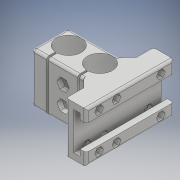
# Autodesk Inventor part: CarroXY - Carro V2
Saved by Autodesk Inventor 2017 (Build 210142000, 142)
## iProperties
Created: 2020-08-15
Part Number: CarroXY - Carro V2
Material: Generic
Document SubType Name: Modeling
Designer: ale
Density: 1 g/cm^3
Appearance: Default
Author: ale
Autodesk Inventor part; units mm, degrees
ref_plane "YZ Plane" through (0, 0, 0) normal (1, 0, 0) x (0, 1, 0)
ref_plane "XZ Plane" through (0, 0, 0) normal (0, 1, 0) x (-1, 0, 0)
ref_plane "XY Plane" through (0, 0, 0) normal (0, 0, 1) x (1, 0, 0)
sketch "Sketch1" plane through (0, 0, 0) normal (0, 0, 1) x (1, 0, 0)
  arc A0 (-11.7683, -9.9732) -> (-13.2317, -9.9732) centre (-12.5, 0) ccw
  arc A1 (13.2317, -9.9732) -> (11.7683, -9.9732) centre (12.5, 0) ccw
  line L0 (23, -17) -> (23, 12)
  line L1 (23, 12) -> (-25, 12)
  line L2 (-25, 12) -> (-25, -17)
  line L3 (-13.2317, -9.9732) -> (-13.2317, -17)
  line L4 (-11.7683, -9.9732) -> (-11.7683, -17)
  line L5 (11.7683, -9.9732) -> (11.7683, -17)
  line L6 (13.2317, -9.9732) -> (13.2317, -17)
  line L7 (13.2317, -17) -> (23, -17)
  line L8 (-25, -17) -> (-13.2317, -17)
  line L9 (-11.7683, -17) -> (11.7683, -17)
  line L10 (-35.4015, 0) -> (35.4015, 0)
  line L11 (0, -27.2768) -> (0, 27.2768)
  point P0 (0, 0)
  point P1 (0, 0)
  point P2 (0, 0)
  dimension "d2" = 20
  dimension "d3" = 20
  dimension "d106" = 17
  dimension "d107" = 17
  dimension "d108" = 17
  dimension "d110" = 12.5
  dimension "d111" = 12.5
  dimension "d113" = 23
  dimension "d114" = 25
  constraints: 24 end point, 4 point on circle, 3 horizontal, 2 centre point, 2 coincident, 2 midpoint, 2 point on line, 1 parallel, 1 vertical
  measures "d2" diameter of A0
  measures "d3" diameter of A1
  measures "d106" distance between parallel lines of L7 L10
  measures "d107" distance between parallel lines of L9 L10
  measures "d108" distance between parallel lines of L8 L10
  measures "d110" distance from line of A1.centre L11
  measures "d111" distance from line of A0.centre L11
  measures "d113" distance between parallel lines of L0 L11
  measures "d114" distance between parallel lines of L2 L11
extrude "Extrusion2" add sketch "Sketch1" along normal blind 40 contours A0 L10 L11 L9 L4 | A0 L10 L2 L1 L11 | A0 L3 L8 L2 L10 | L11 L1 L0 L10 A1 | L10 A1 L5 L9 L11 | L10 L0 L7 L6 A1
sketch "Sketch3" plane through (23, -17, 0) normal (1, 0, 0) x (0, 0, -1)
  line L0 (-40, 49.5) -> (0, 49.5)
  line L1 (0, 49.5) -> (0, -20.5)
  line L2 (0, -20.5) -> (-40, -20.5)
  line L3 (-40, -20.5) -> (-40, 49.5)
  line L4 (-40, 49.5) -> (0, -20.5) construction
  line L5 (0, 49.5) -> (-40, -20.5) construction
  line L6 (0, 29) -> (-40, 29) projected
  line L7 (-20, 29) -> (-20, 0)
  line L8 (0, 0) -> (-40, 0) projected
  line L9 (-40, 0) -> (-40, 29) projected
  line L10 (-40, 14.5) -> (0, 14.5)
  line L11 (0, 29) -> (0, 0) projected
  point P0 (0, 17)
  point P1 (-20, 14.5)
  point P2 (-20, 14.5)
  dimension "d18" = 40
  dimension "d19" = 70
  constraints: 16 end point, 8 midpoint, 2 parallel, 1 horizontal, 1 perpendicular
  measures "d18" distance of L1.end L2.end
  measures "d19" distance between parallel lines of L2 L0
extrude "Extrusion3" add sketch "Sketch3" along normal blind 6
sketch "Sketch13" plane through (-25, 12, 40) normal (0, 1, 0) x (1, 0, 0)
  line L0 (25, 40) -> (25, 0)
  line L1 (13.2317, 0) -> (36.7683, 0) projected
  line L2 (25, 40) -> (65, 40) construction
  line L3 (25, 20) -> (32.3928, 20)
  line L4 (25, 27.5) -> (32.3928, 27.5)
  line L5 (25, 12.5) -> (32.3928, 12.5)
  dimension "d83" = 90
  dimension "d84" = 7.5
  dimension "d85" = 7.5
  constraints: 10 end point, 2 coincident, 2 horizontal, 2 midpoint, 2 parallel, 1 perpendicular
  measures "d83" angle of L0 L2
  measures "d84" distance between parallel lines of L3 L4
  measures "d85" distance between parallel lines of L3 L5
hole "Hole5" at (0, 12, 12.5) at (0, 12, 27.5) direction (0, -1, 0) diameter 4.5 end through all counterbore diameter 10 counterbore depth 3
sketch "Sketch14" plane through (-11.7683, -17, 0) normal (0, -1, 0) x (1, 0, 0)
  circle A0 centre (11.7683, 12.5) radius 2.25 projected
  circle A1 centre (11.7683, 12.5) radius 5 projected
  line L0 (16.7683, 12.5) -> (14.2683, 8.1699)
  line L1 (14.2683, 8.1699) -> (9.2683, 8.1699)
  line L2 (9.2683, 8.1699) -> (6.7683, 12.5)
  line L3 (6.7683, 12.5) -> (9.2683, 16.8301)
  line L4 (9.2683, 16.8301) -> (14.2683, 16.8301)
  line L5 (14.2683, 16.8301) -> (16.7683, 12.5)
  circle A2 centre (11.7683, 27.5) radius 2.25 projected
  circle A3 centre (11.7683, 27.5) radius 5 projected
  line L6 (9.2683, 31.8301) -> (14.2683, 31.8301)
  line L7 (14.2683, 31.8301) -> (16.7683, 27.5)
  line L8 (16.7683, 27.5) -> (14.2683, 23.1699)
  line L9 (14.2683, 23.1699) -> (9.2683, 23.1699)
  line L10 (9.2683, 23.1699) -> (6.7683, 27.5)
  line L11 (6.7683, 27.5) -> (9.2683, 31.8301)
  point P0 (11.7683, 0)
  constraints: 24 end point, 2 coincident, 1 horizontal alignment, 29 other
extrude "Extrusion11" cut sketch "Sketch14" against normal blind 4 contours L0 L1 L2 L3 L4 L5 | L8 L9 L10 L11 L6 L7
sketch "Sketch16" plane through (23, -37.5, 0) normal (0, -1, 0) x (1, 0, 0)
  line L0 (6, 40) -> (6, 0) projected
  line L1 (6, 0) -> (6, 5)
  line L2 (6, 5) -> (11, 5)
  line L3 (11, 5) -> (11, 10)
  line L4 (11, 10) -> (16, 10)
  line L5 (16, 10) -> (16, 0)
  line L6 (16, 0) -> (6, 0)
  line L7 (6, 20) -> (15.5722, 20)
  line L8 (6, 0) -> (6, 40)
  line L9 (6, 40) -> (6, 35)
  line L10 (6, 35) -> (11, 35)
  line L11 (11, 35) -> (11, 30)
  line L12 (11, 30) -> (16, 30)
  line L13 (16, 30) -> (16, 40)
  line L14 (16, 40) -> (6, 40)
  point P0 (-23, 0)
  dimension "d95" = 5
  dimension "d96" = 5
  dimension "d97" = 5
  dimension "d98" = 5
  constraints: 28 end point, 7 symmetric about line, 5 perpendicular, 2 point on line, 1 horizontal, 1 midpoint
  measures "d95" distance of L0.end L1.end
  measures "d96" distance of L1.end L2.end
  measures "d97" distance of L2.end L3.end
  measures "d98" distance of L3.end L4.end
extrude "Extrusion12" add sketch "Sketch16" against normal blind 70
sketch "Sketch10" plane through (-25, -17, 0) normal (-1, 0, 0) x (0, 0, 1)
  line L0 (0, 0) -> (40, 0) projected
  line L1 (20, 0) -> (20, 29)
  line L2 (0, 29) -> (40, 29) projected
  point P0 (0, 17)
  point P1 (35.2144, 3.7)
  point P2 (4.7856, 3.7)
  dimension "d61" = 3.7
  constraints: 2 end point, 2 midpoint, 1 symmetric about line
  measures "d61" distance from line of point (35.214, 3.7) L0
hole "Hole3" at (-25, -13.3, 35.2144) at (-25, -13.3, 4.7856) direction (1, 0, 0) diameter 4.5 end through all
sketch "Sketch17" plane through (39, -37.5, 10) normal (1, 0, 0) x (0, 0, -1)
  circle A0 centre (5.2144, 24.2) radius 2.25 projected
  line L0 (5, 0) -> (5, 70) projected
  line L1 (5, 27.7) -> (8.1383, 26.1357)
  line L2 (8.1383, 26.1357) -> (8.3527, 22.6357)
  line L3 (8.3527, 22.6357) -> (5.4289, 20.7)
  line L4 (5.4289, 20.7) -> (2.2906, 22.2643)
  line L5 (2.2906, 22.2643) -> (2.0761, 25.7643)
  line L6 (2.0761, 25.7643) -> (5, 27.7)
  circle A1 centre (-25.2144, 24.2) radius 2.25 projected
  line L7 (-25, 70) -> (-25, 26.4398) projected
  line L8 (-25, 27.7) -> (-22.0761, 25.7643)
  line L9 (-22.0761, 25.7643) -> (-22.2906, 22.2643)
  line L10 (-22.2906, 22.2643) -> (-25.4289, 20.7)
  line L11 (-25.4289, 20.7) -> (-28.3527, 22.6357)
  line L12 (-28.3527, 22.6357) -> (-28.1383, 26.1357)
  line L13 (-28.1383, 26.1357) -> (-25, 27.7)
  point P0 (10, 37.5)
  point P1 (5.2144, 24.2)
  point P2 (-25.2144, 24.2)
  dimension "d101" = 7
  dimension "d102" = 7
  constraints: 24 end point, 2 coincident, 2 point on line, 27 other
  measures "d101" vertical distance of L1.start L3.end
  measures "d102" vertical distance of L8.start L10.end
extrude "Extrusion13" cut sketch "Sketch17" against normal blind 20 contours A0 L0 L1 L2 L3 L4 | A0 L0 L4 L5 L6 | L8 L9 L10 L11 L12 L13
fillet "Fillet2" radius 2 20 edges at (-25, -17, 20) (-19.1159, -17, 0) (0, -17, 0) (18.1159, -17, 0) (-1, 12, 0) (-25, -2.5, 0) (-25, 12, 20) (-1, 12, 40) (-25, -2.5, 40) (-19.1159, -17, 40) (0, -17, 40) (18.1159, -17, 40) (23, -37.5, 20) (39, -37.5, 5) (39, -37.5, 35) (39, -2.5, 0) (39, -2.5, 40) (23, 32.5, 20) (39, 32.5, 35) (39, 32.5, 5)
sketch "Sketch18" plane through (23, -17, 0) normal (-1, 0, 0) x (0, 0, 1)
  line L0 (40, -18.5) -> (40, 2) projected
  line L1 (2, 0) -> (38, 0) projected
  line L2 (40, -18.5) -> (0, -18.5) projected
  line L3 (20, -18.5) -> (20, -3.6839)
  line L4 (40, 2) -> (40, 27) projected
  line L5 (40, 14.5) -> (0, 14.5)
  point P0 (0, 17)
  point P1 (34.5, -10.25)
  point P2 (5.5, -10.25)
  point P3 (34.5, 39.25)
  point P4 (5.5, 39.25)
  dimension "d119" = 5.5
  dimension "d120" = 10.25
  constraints: 4 end point, 3 symmetric about line, 2 midpoint, 1 horizontal, 1 vertical
  measures "d119" distance from line of L0 point (34.5, -10.25)
  measures "d120" distance from line of L1 point (34.5, -10.25)
chamfer "Chamfer2" distance 7 angle 45 6 edges at (23, -17, 20) (23, -16.4142, 39.4142) (23, -16.4142, 0.5858) (23, 12, 20) (23, 11.4142, 39.4142) (23, 11.4142, 0.5858)
hole "Hole6" at (23, -27.25, 34.5) at (23, -27.25, 5.5) at (23, 22.25, 34.5) at (23, 22.25, 5.5) direction (1, 0, 0) diameter 4.5 end through all
sketch "Sketch19" plane through (39, -35.5, 10) normal (1, 0, 0) x (0, 0, -1)
  circle A0 centre (4.5, 8.25) radius 2.25 projected
  line L0 (4.5, 11.75) -> (7.5311, 10)
  line L1 (7.5311, 10) -> (7.5311, 6.5)
  line L2 (7.5311, 6.5) -> (4.5, 4.75)
  line L3 (4.5, 4.75) -> (1.4689, 6.5)
  line L4 (1.4689, 6.5) -> (1.4689, 10)
  line L5 (1.4689, 10) -> (4.5, 11.75)
  line L6 (-25, -2) -> (5, -2) projected
  line L7 (-10, -2) -> (-10, 68)
  circle A1 centre (-24.5, 8.25) radius 2.25
  line L8 (-24.5, 11.75) -> (-27.5311, 10)
  line L9 (-27.5311, 10) -> (-27.5311, 6.5)
  line L10 (-27.5311, 6.5) -> (-24.5, 4.75)
  line L11 (-24.5, 4.75) -> (-21.4689, 6.5)
  line L12 (-21.4689, 6.5) -> (-21.4689, 10)
  line L13 (-21.4689, 10) -> (-24.5, 11.75)
  circle A2 centre (4.5, 57.75) radius 2.25 projected
  line L14 (4.5, 61.25) -> (7.5311, 59.5)
  line L15 (7.5311, 59.5) -> (7.5311, 56)
  line L16 (7.5311, 56) -> (4.5, 54.25)
  line L17 (4.5, 54.25) -> (1.4689, 56)
  line L18 (1.4689, 56) -> (1.4689, 59.5)
  line L19 (1.4689, 59.5) -> (4.5, 61.25)
  circle A3 centre (-24.5, 57.75) radius 2.25
  line L20 (-24.5, 61.25) -> (-27.5311, 59.5)
  line L21 (-27.5311, 59.5) -> (-27.5311, 56)
  line L22 (-27.5311, 56) -> (-24.5, 54.25)
  line L23 (-24.5, 54.25) -> (-21.4689, 56)
  line L24 (-21.4689, 56) -> (-21.4689, 59.5)
  line L25 (-21.4689, 59.5) -> (-24.5, 61.25)
  dimension "d128" = 7
  dimension "d129" = 7
  constraints: 50 end point, 16 symmetric about line, 4 coincident, 2 centre point, 1 midpoint, 28 other
  measures "d128" distance of L0.start L2.end
  measures "d129" distance of L14.start L16.end
extrude "Extrusion14" cut sketch "Sketch19" against normal blind 13
body "Solid2"
